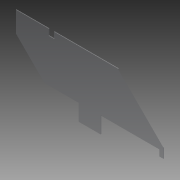
# Autodesk Inventor part: Pneumatics Board
Saved by Autodesk Inventor 2014 (Build 180170000, 170)
## iProperties
Created: 2014-01-30
Part Number: Pneumatics Board
Material: Polycarbonate, Clear
Document SubType Name: Modeling
Designer: Andrew Toennies
Mass: 595.926 g
Surface Area: 3193.54 cm^2
Volume: 496.605 cm^3
Density: 1.2 g/cm^3
Appearance: Polycarbonate - Clear
Author: Andrew Toennies
Autodesk Inventor part; units mm, degrees
ref_plane "YZ Plane" through (0, 0, 0) normal (1, 0, 0) x (0, 1, 0)
ref_plane "XZ Plane" through (0, 0, 0) normal (0, 1, 0) x (-1, 0, 0)
ref_plane "XY Plane" through (0, 0, 0) normal (0, 0, 1) x (1, 0, 0)
sketch "Sketch1" plane through (0, 0, 0) normal (0, 0, 1) x (1, 0, 0)
  line L0 (0, 0) -> (0, -257.175)
  line L1 (0, -257.175) -> (19.05, -257.175)
  line L2 (19.05, -257.175) -> (19.05, -228.6)
  line L3 (666.75, -228.6) -> (666.75, -257.175)
  line L4 (666.75, -257.175) -> (685.8, -257.175)
  line L5 (685.8, -257.175) -> (685.8, 0)
  line L6 (152.4, 0) -> (152.4, -28.575)
  line L7 (152.4, -28.575) -> (177.8, -28.575)
  line L8 (177.8, -28.575) -> (177.8, 0)
  line L9 (0, 0) -> (152.4, 0)
  line L10 (508, 0) -> (508, -28.575)
  line L11 (508, -28.575) -> (533.4, -28.575)
  line L12 (533.4, -28.575) -> (533.4, 0)
  line L13 (177.8, 0) -> (508, 0)
  line L14 (533.4, 0) -> (685.8, 0)
  line L15 (292.1, -228.6) -> (292.1, -304.8)
  line L16 (292.1, -304.8) -> (393.7, -304.8)
  line L17 (393.7, -304.8) -> (393.7, -228.6)
  line L18 (19.05, -228.6) -> (292.1, -228.6)
  line L19 (393.7, -228.6) -> (666.75, -228.6)
  dimension "d0" = 685.8
  dimension "d1" = 257.175
  dimension "d2" = 19.05
  dimension "d3" = 28.575
  dimension "d4" = 28.575
  dimension "d5" = 19.05
  dimension "d6" = 28.575
  dimension "d7" = 25.4
  dimension "d8" = 152.4
  dimension "d9" = 152.4
  dimension "d12" = 76.2
  dimension "d13" = 101.6
  dimension "d14" = 292.1
  constraints: 40 end point, 16 perpendicular, 10 parallel, 3 collinear, 3 equal length, 3 horizontal
  measures "d0" distance of L0.start L5.end
  measures "d1" distance of L0.start L0.end
  measures "d2" distance of L0.end L1.end
  measures "d3" distance of L1.end L2.end
  measures "d4" distance of L3.start L3.end
  measures "d5" distance of L3.end L4.end
  measures "d6" distance of L6.start L6.end
  measures "d7" distance of L6.end L7.end
  measures "d8" distance between parallel lines of L5 L12
  measures "d9" distance between parallel lines of L0 L6
  measures "d12" distance of L15.start L15.end
  measures "d13" distance of L15.end L16.end
  measures "d14" distance between parallel lines of L5 L17
extrude "Extrusion1" add sketch "Sketch1" along normal blind 3.175
sketch "Sketch2" plane through (0, 0, 3.175) normal (0, 0, 1) x (1, 0, 0)
  circle A0 centre (579.273, -176.4988) radius 2.3812 projected
  circle A1 centre (612.547, -176.4988) radius 2.3812 projected
  circle A2 centre (612.547, -210.8512) radius 2.3812 projected
  circle A3 centre (579.273, -210.8512) radius 2.3812 projected
  line L0 (48.9963, -118.9314) -> (48.9963, -129.4314) projected
  line L1 (48.9963, -129.4314) -> (44.9963, -133.7314) projected
  line L2 (44.9963, -133.7314) -> (44.9963, -189.1314) projected
  line L3 (44.9963, -189.1314) -> (48.9963, -193.4314) projected
  line L4 (48.9963, -193.4314) -> (48.9963, -207.5314) projected
  arc A4 (48.9963, -207.5314) -> (50.9963, -209.5314) centre (50.9963, -207.5314) ccw projected
  line L5 (50.9963, -209.5314) -> (59.3463, -209.5314) projected
  line L6 (59.3463, -200.0314) -> (59.3463, -209.5314) projected
  line L7 (56.3963, -200.0314) -> (59.3463, -200.0314) projected
  line L8 (56.3963, -129.4314) -> (56.3963, -200.0314) projected
  line L9 (59.3463, -129.4314) -> (56.3963, -129.4314) projected
  line L10 (59.3463, -116.9314) -> (59.3463, -129.4314) projected
  line L11 (59.3463, -116.9314) -> (50.9963, -116.9314) projected
  arc A5 (50.9963, -116.9314) -> (48.9963, -118.9314) centre (50.9963, -118.9314) ccw projected
  arc A6 (57.7963, -204.9314) -> (53.1963, -204.9314) centre (55.4963, -204.9314) ccw projected
  arc A7 (53.1963, -204.9314) -> (57.7963, -204.9314) centre (55.4963, -204.9314) ccw projected
  arc A8 (57.7963, -121.9314) -> (53.1963, -121.9314) centre (55.4963, -121.9314) ccw projected
  arc A9 (53.1963, -121.9314) -> (57.7963, -121.9314) centre (55.4963, -121.9314) ccw projected
  arc A10 (181.4963, -202.4314) -> (181.4963, -207.4314) centre (181.4963, -204.9314) ccw projected
  line L12 (182.9963, -202.4314) -> (181.4963, -202.4314) projected
  arc A11 (185.4963, -204.9314) -> (182.9963, -202.4314) centre (182.9963, -204.9314) ccw projected
  arc A12 (182.9963, -207.4314) -> (185.4963, -204.9314) centre (182.9963, -204.9314) ccw projected
  line L13 (181.4963, -207.4314) -> (182.9963, -207.4314) projected
  arc A13 (181.4963, -119.4314) -> (181.4963, -124.4314) centre (181.4963, -121.9314) ccw projected
  line L14 (182.9963, -119.4314) -> (181.4963, -119.4314) projected
  arc A14 (185.4963, -121.9314) -> (182.9963, -119.4314) centre (182.9963, -121.9314) ccw projected
  arc A15 (182.9963, -124.4314) -> (185.4963, -121.9314) centre (182.9963, -121.9314) ccw projected
  line L15 (181.4963, -124.4314) -> (182.9963, -124.4314) projected
  line L16 (177.6463, -129.4314) -> (177.6463, -116.9314) projected
  line L17 (181.9963, -129.4314) -> (177.6463, -129.4314) projected
  line L18 (181.9963, -200.0314) -> (181.9963, -129.4314) projected
  line L19 (177.6463, -200.0314) -> (181.9963, -200.0314) projected
  line L20 (177.6463, -209.5314) -> (177.6463, -200.0314) projected
  line L21 (177.6463, -209.5314) -> (185.4963, -209.5314) projected
  arc A16 (185.4963, -209.5314) -> (187.4963, -207.5314) centre (185.4963, -207.5314) ccw projected
  line L22 (187.4963, -207.5314) -> (187.4963, -118.9314) projected
  arc A17 (187.4963, -118.9314) -> (185.4963, -116.9314) centre (185.4963, -118.9314) ccw projected
  line L23 (185.4963, -116.9314) -> (177.6463, -116.9314) projected
  line L24 (93.9565, -45.8769) -> (93.9565, -27.8769) projected
  arc A18 (93.9565, -27.8769) -> (89.9565, -23.8769) centre (89.9565, -27.8769) ccw projected
  line L25 (89.9565, -23.8769) -> (59.9565, -23.8769) projected
  arc A19 (59.9565, -23.8769) -> (55.9565, -27.8769) centre (59.9565, -27.8769) ccw projected
  line L26 (55.9565, -27.8769) -> (55.9565, -45.8769) projected
  line L27 (93.9565, -45.8769) -> (55.9565, -45.8769) projected
  line L28 (63.3065, -43.0869) -> (70.8065, -43.0869) projected
  arc A20 (63.3065, -37.5869) -> (63.3065, -43.0869) centre (63.3065, -40.3369) ccw projected
  line L29 (70.8065, -37.5869) -> (63.3065, -37.5869) projected
  arc A21 (70.8065, -43.0869) -> (70.8065, -37.5869) centre (70.8065, -40.3369) ccw projected
  line L30 (79.3065, -35.1269) -> (86.8065, -35.1269) projected
  arc A22 (79.3065, -29.6269) -> (79.3065, -35.1269) centre (79.3065, -32.3769) ccw projected
  line L31 (86.8065, -29.6269) -> (79.3065, -29.6269) projected
  arc A23 (86.8065, -35.1269) -> (86.8065, -29.6269) centre (86.8065, -32.3769) ccw projected
  line L32 (323.95, -276.45) -> (323.95, -294.45) projected
  arc A24 (323.95, -294.45) -> (327.95, -298.45) centre (327.95, -294.45) ccw projected
  line L33 (327.95, -298.45) -> (357.95, -298.45) projected
  arc A25 (357.95, -298.45) -> (361.95, -294.45) centre (357.95, -294.45) ccw projected
  line L34 (361.95, -294.45) -> (361.95, -276.45) projected
  line L35 (323.95, -276.45) -> (361.95, -276.45) projected
  line L36 (354.6, -279.24) -> (347.1, -279.24) projected
  arc A26 (354.6, -284.74) -> (354.6, -279.24) centre (354.6, -281.99) ccw projected
  line L37 (347.1, -284.74) -> (354.6, -284.74) projected
  arc A27 (347.1, -279.24) -> (347.1, -284.74) centre (347.1, -281.99) ccw projected
  line L38 (338.6, -287.2) -> (331.1, -287.2) projected
  arc A28 (338.6, -292.7) -> (338.6, -287.2) centre (338.6, -289.95) ccw projected
  line L39 (331.1, -292.7) -> (338.6, -292.7) projected
  arc A29 (331.1, -287.2) -> (331.1, -292.7) centre (331.1, -289.95) ccw projected
  circle A30 centre (503, -189.9) radius 3.5 projected
  circle A31 centre (447.0388, -189.9) radius 3.5177 projected
  constraints: 1 other
extrude "Extrusion2" cut sketch "Sketch2" against normal blind 25.4 contours A0 | A1 | A2 | A3 | A7 A6 | A9 A8 | L12 A11 A12 L13 A10 | L14 A14 A15 L15 A13 | A20 L29 A21 L28 | A22 L31 A23 L30 | A26 L37 A27 L36 | A28 L39 A29 L38 | A30 | A31
sketch "Sketch3" plane through (0, 0, 3.175) normal (0, 0, 1) x (1, 0, 0)
  line L0 (19.05, -228.6) -> (292.1, -228.6) projected
  line L1 (393.7, -228.6) -> (666.75, -228.6) projected
  line L2 (508, -28.575) -> (508, 0) projected
  line L3 (508, 0) -> (177.8, 0) projected
  line L4 (431.8, -25.4) -> (457.2, -25.4)
  line L5 (457.2, -25.4) -> (457.2, -31.75)
  line L6 (457.2, -31.75) -> (431.8, -31.75)
  line L7 (431.8, -31.75) -> (431.8, -25.4)
  line L8 (279.4, -215.9) -> (304.8, -215.9)
  line L9 (304.8, -215.9) -> (304.8, -222.25)
  line L10 (304.8, -222.25) -> (279.4, -222.25)
  line L11 (279.4, -222.25) -> (279.4, -215.9)
  line L12 (381, -215.9) -> (406.4, -215.9)
  line L13 (406.4, -215.9) -> (406.4, -222.25)
  line L14 (406.4, -222.25) -> (381, -222.25)
  line L15 (381, -222.25) -> (381, -215.9)
  circle A0 centre (55.4963, -204.9314) radius 2.3 projected
  arc A1 (347.1, -279.24) -> (347.1, -284.74) centre (347.1, -281.99) ccw projected
  line L16 (347.1, -279.24) -> (354.6, -279.24) projected
  arc A2 (354.6, -284.74) -> (354.6, -279.24) centre (354.6, -281.99) ccw projected
  line L17 (354.6, -284.74) -> (347.1, -284.74) projected
  arc A3 (70.8065, -43.0869) -> (70.8065, -37.5869) centre (70.8065, -40.3369) ccw projected
  line L18 (70.8065, -43.0869) -> (63.3065, -43.0869) projected
  arc A4 (63.3065, -37.5869) -> (63.3065, -43.0869) centre (63.3065, -40.3369) ccw projected
  line L19 (63.3065, -37.5869) -> (70.8065, -37.5869) projected
  line L20 (182.9963, -207.4314) -> (181.4963, -207.4314) projected
  arc A5 (181.4963, -202.4314) -> (181.4963, -207.4314) centre (181.4963, -204.9314) ccw projected
  line L21 (181.4963, -202.4314) -> (182.9963, -202.4314) projected
  arc A6 (182.9963, -207.4314) -> (182.9963, -202.4314) centre (182.9963, -204.9314) ccw projected
  circle A7 centre (503, -189.9) radius 3.5 projected
  circle A8 centre (612.547, -210.8512) radius 2.3812 projected
  circle A9 centre (579.273, -176.4988) radius 2.3812 projected
  circle A10 centre (612.547, -176.4988) radius 2.3812 projected
  circle A11 centre (579.273, -210.8512) radius 2.3812 projected
  circle A12 centre (447.0388, -189.9) radius 3.5177 projected
  line L22 (182.9963, -124.4314) -> (181.4963, -124.4314) projected
  arc A13 (181.4963, -119.4314) -> (181.4963, -124.4314) centre (181.4963, -121.9314) ccw projected
  line L23 (181.4963, -119.4314) -> (182.9963, -119.4314) projected
  arc A14 (182.9963, -124.4314) -> (182.9963, -119.4314) centre (182.9963, -121.9314) ccw projected
  arc A15 (86.8065, -35.1269) -> (86.8065, -29.6269) centre (86.8065, -32.3769) ccw projected
  line L24 (86.8065, -35.1269) -> (79.3065, -35.1269) projected
  arc A16 (79.3065, -29.6269) -> (79.3065, -35.1269) centre (79.3065, -32.3769) ccw projected
  line L25 (79.3065, -29.6269) -> (86.8065, -29.6269) projected
  arc A17 (331.1, -287.2) -> (331.1, -292.7) centre (331.1, -289.95) ccw projected
  line L26 (331.1, -287.2) -> (338.6, -287.2) projected
  arc A18 (338.6, -292.7) -> (338.6, -287.2) centre (338.6, -289.95) ccw projected
  line L27 (338.6, -292.7) -> (331.1, -292.7) projected
  circle A19 centre (55.4963, -121.9314) radius 2.3 projected
  line L28 (0, 0) -> (0, -257.175) projected
  line L29 (0, -257.175) -> (19.05, -257.175) projected
  line L30 (19.05, -257.175) -> (19.05, -228.6) projected
  line L31 (19.05, -228.6) -> (292.1, -228.6) projected
  line L32 (292.1, -228.6) -> (292.1, -304.8) projected
  line L33 (292.1, -304.8) -> (393.7, -304.8) projected
  line L34 (393.7, -304.8) -> (393.7, -228.6) projected
  line L35 (393.7, -228.6) -> (666.75, -228.6) projected
  line L36 (666.75, -228.6) -> (666.75, -257.175) projected
  line L37 (666.75, -257.175) -> (685.8, -257.175) projected
  line L38 (685.8, -257.175) -> (685.8, 0) projected
  line L39 (685.8, 0) -> (533.4, 0) projected
  line L40 (533.4, 0) -> (533.4, -28.575) projected
  line L41 (533.4, -28.575) -> (508, -28.575) projected
  line L42 (508, -28.575) -> (508, 0) projected
  line L43 (508, 0) -> (177.8, 0) projected
  line L44 (177.8, 0) -> (177.8, -28.575) projected
  line L45 (177.8, -28.575) -> (152.4, -28.575) projected
  line L46 (152.4, -28.575) -> (152.4, 0) projected
  line L47 (152.4, 0) -> (0, 0) projected
  line L48 (207.1624, -63.5) -> (192.9003, -63.5)
  line L49 (207.1624, -63.5) -> (192.9003, -63.5)
  ellipse E0 centre (219.075, -318.5775) end of major axis (222.4532, -318.5775) minor radius 3.3649 (215.9762, -319.9174) -> (215.9762, -317.2376) ccw projected
  line L50 (215.9762, -325.895) -> (215.9762, -319.9174) projected
  ellipse E1 centre (215.9, -327.9555) end of major axis (213.8299, -327.9555) minor radius 2.0619 (215.9762, -330.016) -> (215.9762, -325.895) ccw projected
  line L51 (215.9762, -351.1947) -> (215.9762, -330.016) projected
  ellipse E2 centre (215.9, -353.2552) end of major axis (213.8299, -353.2552) minor radius 2.0619 (215.9762, -355.3158) -> (215.9762, -351.1947) ccw projected
  line L52 (215.9762, -376.4945) -> (215.9762, -355.3158) projected
  ellipse E3 centre (215.9, -378.555) end of major axis (213.8299, -378.555) minor radius 2.0619 (215.9762, -380.6155) -> (215.9762, -376.4945) ccw projected
  line L53 (215.9762, -401.7942) -> (215.9762, -380.6155) projected
  ellipse E4 centre (215.9, -403.8548) end of major axis (213.8299, -403.8548) minor radius 2.0619 (215.9762, -405.9153) -> (215.9762, -401.7942) ccw projected
  line L54 (215.9762, -427.094) -> (215.9762, -405.9153) projected
  ellipse E5 centre (215.9, -429.1545) end of major axis (213.8299, -429.1545) minor radius 2.0619 (215.9762, -431.215) -> (215.9762, -427.094) ccw projected
  line L55 (215.9762, -452.3937) -> (215.9762, -431.215) projected
  ellipse E6 centre (215.9, -454.4543) end of major axis (213.8299, -454.4543) minor radius 2.0619 (215.9762, -456.5148) -> (215.9762, -452.3937) ccw projected
  line L56 (215.9762, -477.6935) -> (215.9762, -456.5148) projected
  ellipse E7 centre (215.9, -479.754) end of major axis (213.8299, -479.754) minor radius 2.0619 (215.9762, -481.8146) -> (215.9762, -477.6935) ccw projected
  line L57 (215.9762, -502.9932) -> (215.9762, -481.8146) projected
  ellipse E8 centre (215.9, -505.0538) end of major axis (213.8299, -505.0538) minor radius 2.0619 (215.9762, -507.1143) -> (215.9762, -502.9932) ccw projected
  line L58 (215.9762, -528.293) -> (215.9762, -507.1143) projected
  ellipse E9 centre (215.9, -530.3535) end of major axis (213.8299, -530.3535) minor radius 2.0619 (215.9762, -532.4141) -> (215.9762, -528.293) ccw projected
  line L59 (215.9762, -553.5927) -> (215.9762, -532.4141) projected
  ellipse E10 centre (215.9, -555.6533) end of major axis (213.8299, -555.6533) minor radius 2.0619 (215.9762, -557.7138) -> (215.9762, -553.5927) ccw projected
  line L60 (215.9762, -578.8925) -> (215.9762, -557.7138) projected
  ellipse E11 centre (215.9, -580.953) end of major axis (213.8299, -580.953) minor radius 2.0619 (215.9762, -583.0136) -> (215.9762, -578.8925) ccw projected
  line L61 (215.9762, -604.1923) -> (215.9762, -583.0136) projected
  ellipse E12 centre (215.9, -606.2528) end of major axis (213.8299, -606.2528) minor radius 2.0619 (215.9762, -608.3133) -> (215.9762, -604.1923) ccw projected
  line L62 (215.9762, -629.492) -> (215.9762, -608.3133) projected
  ellipse E13 centre (215.9, -631.5525) end of major axis (213.8299, -631.5525) minor radius 2.0619 (215.9762, -633.6131) -> (215.9762, -629.492) ccw projected
  line L63 (215.9762, -654.7918) -> (215.9762, -633.6131) projected
  ellipse E14 centre (215.9, -656.8523) end of major axis (213.8299, -656.8523) minor radius 2.0619 (215.9762, -658.9128) -> (215.9762, -654.7918) ccw projected
  line L64 (215.9762, -680.0915) -> (215.9762, -658.9128) projected
  ellipse E15 centre (215.9, -682.1521) end of major axis (213.8299, -682.1521) minor radius 2.0619 (217.9701, -682.1521) -> (215.9762, -680.0915) ccw projected
  line L65 (217.9701, -682.1521) -> (228.6, -682.1521) projected
  line L66 (228.6, -62.3081) -> (228.6, -682.1521) projected
  line L67 (215.9762, -62.3081) -> (228.6, -62.3081) projected
  line L68 (215.9762, -72.8974) -> (215.9762, -62.3081) projected
  ellipse E16 centre (215.9, -74.958) end of major axis (213.8299, -74.958) minor radius 2.0619 (215.9762, -77.0185) -> (215.9762, -72.8974) ccw projected
  line L69 (215.9762, -98.1972) -> (215.9762, -77.0185) projected
  ellipse E17 centre (215.9, -100.2577) end of major axis (213.8299, -100.2577) minor radius 2.0619 (215.9762, -102.3182) -> (215.9762, -98.1972) ccw projected
  line L70 (215.9762, -123.4969) -> (215.9762, -102.3182) projected
  ellipse E18 centre (215.9, -125.5575) end of major axis (213.8299, -125.5575) minor radius 2.0619 (215.9762, -127.618) -> (215.9762, -123.4969) ccw projected
  line L71 (215.9762, -148.7967) -> (215.9762, -127.618) projected
  ellipse E19 centre (215.9, -150.8572) end of major axis (213.8299, -150.8572) minor radius 2.0619 (215.9762, -152.9177) -> (215.9762, -148.7967) ccw projected
  line L72 (215.9762, -174.0964) -> (215.9762, -152.9177) projected
  ellipse E20 centre (215.9, -176.157) end of major axis (213.8299, -176.157) minor radius 2.0619 (215.9762, -178.2175) -> (215.9762, -174.0964) ccw projected
  line L73 (215.9762, -199.3962) -> (215.9762, -178.2175) projected
  ellipse E21 centre (215.9, -201.4567) end of major axis (213.8299, -201.4567) minor radius 2.0619 (215.9762, -203.5173) -> (215.9762, -199.3962) ccw projected
  line L74 (215.9762, -224.6959) -> (215.9762, -203.5173) projected
  ellipse E22 centre (215.9, -226.7565) end of major axis (213.8299, -226.7565) minor radius 2.0619 (215.9762, -228.817) -> (215.9762, -224.6959) ccw projected
  line L75 (215.9762, -249.9957) -> (215.9762, -228.817) projected
  ellipse E23 centre (215.9, -252.0562) end of major axis (213.8299, -252.0562) minor radius 2.0619 (215.9762, -254.1168) -> (215.9762, -249.9957) ccw projected
  line L76 (215.9762, -275.2955) -> (215.9762, -254.1168) projected
  ellipse E24 centre (215.9, -277.356) end of major axis (213.8299, -277.356) minor radius 2.0619 (215.9762, -279.4165) -> (215.9762, -275.2955) ccw projected
  line L77 (215.9762, -291.9378) -> (215.9762, -279.4165) projected
  ellipse E25 centre (219.075, -293.2777) end of major axis (222.4532, -293.2777) minor radius 3.3649 (215.9762, -294.6177) -> (215.9762, -291.9378) ccw projected
  line L78 (215.9762, -300.5952) -> (215.9762, -294.6177) projected
  ellipse E26 centre (215.9, -302.6557) end of major axis (213.8299, -302.6557) minor radius 2.0619 (215.9762, -304.7163) -> (215.9762, -300.5952) ccw projected
  line L79 (215.9762, -317.2376) -> (215.9762, -304.7163) projected
  line L80 (207.1624, -115.8748) -> (192.9003, -115.8748)
  line L81 (270.6624, -181.8262) -> (262.7376, -181.8262)
  line L82 (270.6624, -168.2496) -> (256.4003, -168.2496)
  line L83 (279.4, -165.0746) -> (304.8, -165.0746)
  line L84 (304.8, -165.0746) -> (304.8, -171.4246)
  line L85 (304.8, -171.4246) -> (279.4, -171.4246)
  line L86 (279.4, -171.4246) -> (279.4, -165.0746)
  line L87 (381, -165.0746) -> (406.4, -165.0746)
  line L88 (406.4, -165.0746) -> (406.4, -171.4246)
  line L89 (406.4, -171.4246) -> (381, -171.4246)
  line L90 (381, -171.4246) -> (381, -165.0746)
  line L91 (279.4, -112.6998) -> (304.8, -112.6998)
  line L92 (304.8, -112.6998) -> (304.8, -119.0498)
  line L93 (304.8, -119.0498) -> (279.4, -119.0498)
  line L94 (279.4, -119.0498) -> (279.4, -112.6998)
  line L95 (381, -112.6998) -> (406.4, -112.6998)
  line L96 (406.4, -112.6998) -> (406.4, -119.0498)
  line L97 (406.4, -119.0498) -> (381, -119.0498)
  line L98 (381, -119.0498) -> (381, -112.6998)
  line L99 (279.4, -60.325) -> (304.8, -60.325)
  line L100 (304.8, -60.325) -> (304.8, -66.675)
  line L101 (304.8, -66.675) -> (279.4, -66.675)
  line L102 (279.4, -66.675) -> (279.4, -60.325)
  line L103 (381, -60.325) -> (406.4, -60.325)
  line L104 (406.4, -60.325) -> (406.4, -66.675)
  line L105 (406.4, -66.675) -> (381, -66.675)
  line L106 (381, -66.675) -> (381, -60.325)
  line L107 (400.05, -25.4) -> (425.45, -25.4)
  line L108 (425.45, -25.4) -> (425.45, -31.75)
  line L109 (425.45, -31.75) -> (400.05, -31.75)
  line L110 (400.05, -31.75) -> (400.05, -25.4)
  line L111 (342.9, 0) -> (342.9, -77.0185) construction
  line L112 (285.75, -25.4) -> (260.35, -25.4)
  line L113 (260.35, -25.4) -> (260.35, -31.75)
  line L114 (260.35, -31.75) -> (285.75, -31.75)
  line L115 (285.75, -31.75) -> (285.75, -25.4)
  dimension "d17" = 25.4
  dimension "d18" = 6.35
  dimension "d19" = 25.4
  dimension "d20" = 50.8
  dimension "d21" = 6.35
  dimension "d22" = 6.35
  dimension "d23" = 25.4
  dimension "d24" = 25.4
  dimension "d25" = 6.35
  dimension "d26" = 6.35
  dimension "d27" = 50.8
  dimension "d31" = 76.2
  dimension "d33" = 3.175
  dimension "d34" = 3.175
  dimension "d35" = 3.175
  dimension "d76" = 6.35
  dimension "d77" = 25.4
  constraints: 100 end point, 21 parallel, 15 horizontal, 12 equal length, 11 collinear, 10 perpendicular, 4 symmetric about line, 1 midpoint, 37 other
  measures "d17" distance between parallel lines of L5 L7
  measures "d18" distance between parallel lines of L6 L4
  measures "d19" distance between parallel lines of L3 L4
  measures "d20" distance between parallel lines of L2 L5
  measures "d21" distance between parallel lines of L10 L8
  measures "d22" distance between parallel lines of L0 L10
  measures "d23" distance between parallel lines of L9 L11
  measures "d24" distance of L12.start L12.end
  measures "d25" distance of L14.end L12.start
  measures "d26" distance between parallel lines of L1 L14
  measures "d27" distance between parallel lines of L5 L13
  measures "d31" distance between parallel lines of L15 L9
  measures "d33" distance between parallel lines of L82 L85
  measures "d34" distance between parallel lines of L80 L91
  measures "d35" distance between parallel lines of L48 L99
  measures "d76" distance between parallel lines of L7 L108
  measures "d77" distance of L107.start L107.end
extrude "Extrusion4" cut sketch "Sketch3" against normal blind 25.4 contours L8 L9 L10 L11 | L12 L13 L14 L15 | L83 L84 L85 L86 | L87 L88 L89 L90 | L91 L92 L93 L94 | L95 L96 L97 L98 | L99 L100 L101 L102 | L103 L104 L105 L106 | L107 L108 L109 L110 | L115 L114 L113 L112
sketch "Sketch4" plane through (0, 0, 3.175) normal (0, 0, 1) x (1, 0, 0)
  line L0 (508, -28.575) -> (508, 0) projected
  line L1 (508, 0) -> (177.8, 0) projected
  line L2 (152.4, 0) -> (0, 0) projected
  line L3 (298.45, 0) -> (298.45, -31.75)
  line L4 (298.45, -31.75) -> (330.2, -31.75)
  line L5 (330.2, -31.75) -> (330.2, -82.55)
  line L6 (330.2, -82.55) -> (355.6, -82.55)
  line L7 (355.6, -82.55) -> (355.6, -31.75)
  line L8 (355.6, -31.75) -> (387.35, -31.75)
  line L9 (387.35, -31.75) -> (387.35, 0)
  dimension "d38" = 31.75
  dimension "d39" = 31.75
  dimension "d40" = 50.8
  dimension "d41" = 25.4
  dimension "d42" = 50.8
  dimension "d43" = 31.75
  dimension "d44" = 120.65
  constraints: 14 end point, 4 perpendicular, 3 parallel, 2 point on line
  measures "d38" distance of L3.end L3.start
  measures "d39" distance of L3.end L4.end
  measures "d40" distance of L4.end L5.end
  measures "d41" distance of L5.end L6.end
  measures "d42" distance of L6.end L7.end
  measures "d43" distance of L7.end L8.end
  measures "d44" distance between parallel lines of L0 L9
extrude "Extrusion5" cut sketch "Sketch4" against normal blind 25.4
sketch "Sketch5" plane through (0, 0, 3.175) normal (0, 0, 1) x (1, 0, 0)
  line L0 (355.6, -31.75) -> (355.6, -82.55) projected
  arc A0 (342.9762, -90.9687) -> (342.9762, -86.8313) centre (342.9, -88.9) ccw projected
  circle A1 centre (342.9, -88.9) radius 2.0701
  circle A2 centre (342.9, -114.3) radius 2.0701
  circle A3 centre (342.9, -139.7) radius 2.0701
  circle A4 centre (342.9, -165.1) radius 2.0701
  circle A5 centre (342.9, -190.5) radius 2.0701
  circle A6 centre (342.9, -215.9) radius 2.0701
  dimension "d47" = 4.1402
  dimension "d50" = 25.4
  constraints: 6 centre point, 1 coincident, 1 vertical, 10 other
  measures "d47" diameter of A1
  measures "d50" distance of A1.centre A2.centre
extrude "Extrusion6" cut sketch "Sketch5" against normal blind 25.4
sketch "Sketch6" plane through (0, 0, 3.175) normal (0, 0, 1) x (1, 0, 0)
  line L0 (298.45, 0) -> (177.8, 0) projected
  line L1 (508, 0) -> (387.35, 0) projected
  arc A0 (395.7687, -12.6238) -> (391.6313, -12.6238) centre (393.7, -12.7) ccw projected
  arc A1 (294.1687, -12.6238) -> (290.0313, -12.6238) centre (292.1, -12.7) ccw projected
  circle A2 centre (292.1, -12.7) radius 2.0701
  circle A3 centre (393.7, -12.7) radius 2.0701
  circle A4 centre (419.1, -12.7) radius 2.0701
  circle A5 centre (444.5, -12.7) radius 2.0701
  circle A6 centre (469.9, -12.7) radius 2.0701
  circle A7 centre (495.3, -12.7) radius 2.0701
  circle A8 centre (266.7, -12.7) radius 2.0701
  circle A9 centre (241.3, -12.7) radius 2.0701
  circle A10 centre (215.9, -12.7) radius 2.0701
  circle A11 centre (190.5, -12.7) radius 2.0701
  dimension "d57" = 4.1402
  dimension "d58" = 4.1402
  dimension "d61" = 25.4
  dimension "d68" = 25.4
  constraints: 10 centre point, 2 coincident, 2 horizontal, 16 other
  measures "d57" diameter of A2
  measures "d58" diameter of A3
  measures "d61" distance of A3.centre A4.centre
  measures "d68" distance of A2.centre A8.centre
extrude "Extrusion7" cut sketch "Sketch6" against normal blind 25.4
body "Solid1"
